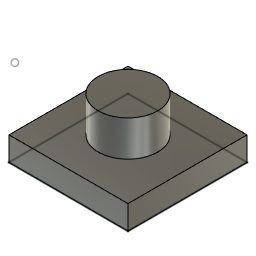
sample (Autodesk Fusion 360 design; units mm, degrees)
Autodesk Fusion 360 part; units mm, degrees
sketch "Sketch1" plane through (0, 0, 0) normal (0, 0, 1) x (1, 0, 0)
  line L0 (-50, 50) -> (50, 50)
  line L1 (50, 50) -> (50, -50)
  line L2 (50, -50) -> (-50, -50)
  line L3 (-50, -50) -> (-50, 50)
  point P0 (-122.6558, 0.4138)
  point P1 (-120, 25)
  dimension "d14" = 100
  dimension "d15" = 100
  dimension "d17" = 50
  dimension "d18" = 50
  constraint horizontal L0
  constraint vertical L1
  constraint horizontal L2
  constraint vertical L3
  measures "d14" distance of L0.start L0.end
  measures "d15" distance of L0.start L2.end
  measures "d17" distance of origin L1
  measures "d18" distance of origin L0
extrude "Extrude1" add sketch "Sketch1" along normal blind 20 makes body 1
sketch "Sketch1 (2)" plane through (0, 0, 0) normal (0, 0, 1) x (1, 0, 0) in component "ChildComponent"
  circle A0 centre (0, 0) radius 25
  dimension "d7" = 50
  constraint coincident A0.centre origin
  measures "d7" diameter of A0
extrude "Extrude1'" add sketch "Sketch1 (2)" along normal blind 30 from surface at 20 separate body makes body 2 in component "ChildComponent"
component "ChildComponent" placed x (1, 0, 0) y (0, 1, 0) z (0, 0, 1) at (0, 0, 0)
equation "modelHeight = 20 mm"
equation "childModelWidth = 50 mm"
equation "d5 = modelHeight"
equation "d7 = childModelWidth"
equation "modelSize = 100 mm"
equation "d14 = modelSize"
equation "d15 = modelSize"
equation "d17 = modelSize / 2"
equation "d18 = modelSize / 2"
